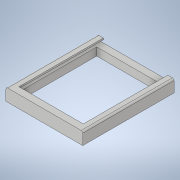
# Autodesk Inventor part: top_bracket_for_5mm
Saved by Autodesk Inventor 2020 (Build 240168000, 168)
## iProperties
Created: 2019-05-08
Part Number: top_bracket_for_5mm
Material: Generic
Document SubType Name: Modeling
Designer: aonih
Density: 1 g/cm^3
Appearance: Default
Author: aonih
Autodesk Inventor part; units mm, degrees
ref_plane "YZ Plane" through (0, 0, 0) normal (1, 0, 0) x (0, 1, 0)
ref_plane "XZ Plane" through (0, 0, 0) normal (0, 1, 0) x (-1, 0, 0)
ref_plane "XY Plane" through (0, 0, 0) normal (0, 0, 1) x (1, 0, 0)
sketch "Sketch1" plane through (0, 0, 0) normal (0, 1, 0) x (-1, 0, 0)
  line L0 (-71.5, -85) -> (71.5, -85)
  line L1 (71.5, -85) -> (71.5, 85)
  line L2 (71.5, 85) -> (-71.5, 85)
  line L3 (-71.5, 85) -> (-71.5, -85)
  line L4 (-71.5, -85) -> (71.5, 85) construction
  line L5 (71.5, -85) -> (-71.5, 85) construction
  point P0 (0, 0)
  dimension "d0" = 143
  dimension "d1" = 170
  constraints: 12 end point, 2 midpoint, 2 parallel, 1 horizontal, 1 perpendicular
  measures "d0" distance of L2.end L1.end
  measures "d1" distance of L1.end L0.end
extrude "Base" add sketch "Sketch1" along normal blind 23
sketch "Sketch2" plane through (0, 0, 0) normal (0, -1, 0) x (1, 0, 0)
  line L0 (-60, -72.5) -> (60, -72.5)
  line L1 (60, -72.5) -> (60, 72.5)
  line L2 (60, 72.5) -> (-60, 72.5)
  line L3 (-60, 72.5) -> (-60, -72.5)
  line L4 (-60, -72.5) -> (60, 72.5) construction
  line L5 (60, -72.5) -> (-60, 72.5) construction
  point P0 (0, 0)
  dimension "d4" = 120
  dimension "d5" = 145
  constraints: 12 end point, 2 midpoint, 2 parallel, 1 horizontal, 1 perpendicular
  measures "d4" distance of L2.end L1.end
  measures "d5" distance of L1.end L0.end
extrude "Extrusion2" cut sketch "Sketch2" against normal through all
sketch "Sketch3" plane through (0, 0, 0) normal (0, -1, 0) x (1, 0, 0)
  line L0 (63.65, -75.5) -> (-63.65, -75.5)
  line L1 (-63.65, -75.5) -> (-63.65, 75.5)
  line L2 (-63.65, 75.5) -> (63.65, 75.5)
  line L3 (63.65, 75.5) -> (63.65, -75.5)
  line L4 (-60, 72.5) -> (60, 72.5) projected
  line L5 (-60, -72.5) -> (-60, 72.5) projected
  line L6 (68.85, -80.7) -> (-68.85, -80.7)
  line L7 (-68.85, -80.7) -> (-68.85, 80.7)
  line L8 (-68.85, 80.7) -> (68.85, 80.7)
  line L9 (68.85, 80.7) -> (68.85, -80.7)
  line L10 (-71.5, 85) -> (71.5, 85) projected
  point P0 (0, 0)
  point P1 (63.65, 0)
  point P2 (68.85, 0)
  dimension "d9" = 3.65
  dimension "d10" = 5.2
  dimension "d11" = 12.5
  dimension "d38" = 5.2
  dimension "d39" = 151
  constraints: 16 end point, 4 parallel, 2 horizontal, 2 horizontal alignment, 2 midpoint, 2 perpendicular
  measures "d9" distance between parallel lines of L5 L1
  measures "d10" distance between parallel lines of L2 L8
  measures "d11" distance between parallel lines of L10 L4
  measures "d38" distance between parallel lines of L3 L9
  measures "d39" distance between parallel lines of L0 L2
extrude "Extrusion3" cut sketch "Sketch3" against normal blind 12
sketch "Sketch4" plane through (0, 12, 0) normal (0, -1, 0) x (1, 0, 0)
  line L0 (-68.85, 80.7) -> (68.85, 80.7) projected
  line L1 (63.65, 75.5) -> (-63.65, 75.5) projected
  line L2 (-53.85, 80.7) -> (-41.85, 80.7)
  line L3 (-41.85, 80.7) -> (-41.85, 75.5)
  line L4 (-41.85, 75.5) -> (-53.85, 75.5)
  line L5 (-53.85, 75.5) -> (-53.85, 80.7)
  line L6 (-68.85, -80.7) -> (-68.85, 80.7) projected
  line L7 (-63.65, 75.5) -> (-63.65, -75.5) projected
  line L8 (-63.65, 66.4) -> (-68.85, 66.4)
  line L9 (-68.85, 66.4) -> (-68.85, 54.4)
  line L10 (-68.85, 54.4) -> (-63.65, 54.4)
  line L11 (-63.65, 54.4) -> (-63.65, 66.4)
  line L12 (63.65, -75.5) -> (63.65, 75.5) projected
  line L13 (68.85, 80.7) -> (68.85, -80.7) projected
  line L14 (63.65, 66.4) -> (68.85, 66.4)
  line L15 (68.85, 66.4) -> (68.85, 54.4)
  line L16 (68.85, 54.4) -> (63.65, 54.4)
  line L17 (63.65, 54.4) -> (63.65, 66.4)
  line L18 (-63.65, -75.5) -> (63.65, -75.5) projected
  line L19 (68.85, -80.7) -> (-68.85, -80.7) projected
  line L20 (-53.85, -75.5) -> (-41.85, -75.5)
  line L21 (-41.85, -75.5) -> (-41.85, -80.7)
  line L22 (-41.85, -80.7) -> (-53.85, -80.7)
  line L23 (-53.85, -80.7) -> (-53.85, -75.5)
  line L24 (-68.85, -66.4) -> (-63.65, -66.4)
  line L25 (-63.65, -66.4) -> (-63.65, -54.4)
  line L26 (-63.65, -54.4) -> (-68.85, -54.4)
  line L27 (-68.85, -54.4) -> (-68.85, -66.4)
  line L28 (53.85, -80.7) -> (41.85, -80.7)
  line L29 (41.85, -80.7) -> (41.85, -75.5)
  line L30 (41.85, -75.5) -> (53.85, -75.5)
  line L31 (53.85, -75.5) -> (53.85, -80.7)
  line L32 (68.85, -54.4) -> (63.65, -54.4)
  line L33 (63.65, -54.4) -> (63.65, -66.4)
  line L34 (63.65, -66.4) -> (68.85, -66.4)
  line L35 (68.85, -66.4) -> (68.85, -54.4)
  line L36 (53.85, 75.5) -> (41.85, 75.5)
  line L37 (41.85, 75.5) -> (41.85, 80.7)
  line L38 (41.85, 80.7) -> (53.85, 80.7)
  line L39 (53.85, 80.7) -> (53.85, 75.5)
  point P0 (0, 0)
  point P1 (66.25, 66.4)
  point P2 (-66.25, 66.4)
  point P3 (-53.85, -78.1)
  point P4 (-53.85, 78.1)
  point P5 (66.25, -54.4)
  point P6 (-66.25, -54.4)
  point P7 (41.85, 78.1)
  point P8 (41.85, -78.1)
  dimension "d14" = 12
  dimension "d15" = 15
  dimension "d16" = 12
  dimension "d17" = 14.3
  dimension "d18" = 12
  dimension "d19" = 12
  dimension "d20" = 14.3
  dimension "d21" = 12
  dimension "d22" = 12
  dimension "d23" = 15
  dimension "d24" = 12
  dimension "d25" = 12
  constraints: 64 end point, 16 parallel, 16 point on line, 8 horizontal, 8 midpoint, 8 perpendicular, 2 horizontal alignment, 2 vertical alignment
  measures "d14" distance between parallel lines of L3 L5
  measures "d15" distance between parallel lines of L6 L5
  measures "d16" distance between parallel lines of L8 L10
  measures "d17" distance between parallel lines of L0 L8
  measures "d18" distance between parallel lines of L14 L16
  measures "d19" distance between parallel lines of L21 L23
  measures "d20" distance between parallel lines of L19 L24
  measures "d21" distance between parallel lines of L26 L24
  measures "d22" distance between parallel lines of L34 L32
  measures "d23" distance between parallel lines of L13 L31
  measures "d24" distance between parallel lines of L31 L29
  measures "d25" distance between parallel lines of L39 L37
extrude "Extrusion4" add sketch "Sketch4" along normal blind 7 contours L0 L3 L1 L5 | L8 L7 L10 L6 | L0 L39 L1 L37 | L26 L7 L24 L6 | L13 L16 L12 L14 | L23 L18 L21 L19 | L13 L34 L12 L32 | L29 L18 L31 L19
fillet "Fillet1" radius 1.25 16 edges at (-66.25, 5, 54.4) (-66.25, 5, 66.4) (-66.25, 5, -66.4) (-66.25, 5, -54.4) (66.25, 5, -66.4) (66.25, 5, -54.4) (66.25, 5, 54.4) (66.25, 5, 66.4) (53.85, 5, -78.1) (41.85, 5, -78.1) (-53.85, 5, -78.1) (-41.85, 5, -78.1) (-53.85, 5, 78.1) (-41.85, 5, 78.1) (41.85, 5, 78.1) (53.85, 5, 78.1)
sketch "Sketch5" plane through (71.5, 0, -85) normal (0, 0, -1) x (-1, 0, 0)
  line L0 (71.5, 0) -> (71.5, 23) construction
  line L1 (131.5, 23) -> (11.5, 23) construction
  line L2 (5, 20.05) -> (138, 20.05)
  line L3 (138, 20.05) -> (138, 14.8)
  line L4 (138, 14.8) -> (5, 14.8)
  line L5 (5, 14.8) -> (5, 20.05)
  line L6 (0, 0) -> (143, 0) projected
  point P0 (71.5, 20.05)
  dimension "d29" = 133
  dimension "d30" = 5.25
  dimension "d31" = 14.8
  constraints: 10 end point, 2 midpoint, 2 parallel, 1 horizontal, 1 perpendicular, 1 point on line
  measures "d29" distance of L3.end L4.end
  measures "d30" distance of L2.end L3.end
  measures "d31" distance between parallel lines of L6 L4
extrude "Extrusion5" cut sketch "Sketch5" against normal blind 165
fillet "Fillet2" radius 3 2 edges at (71.5, 23, 0) (-71.5, 23, 0)
sketch "Sketch6" plane through (71.5, 0, -85) normal (0, 0, -1) x (-1, 0, 0)
  line L0 (3, 23) -> (140, 23) projected
  line L1 (5, 20.05) -> (138, 20.05) projected
  line L2 (11.5, 23) -> (131.5, 23)
  line L3 (131.5, 23) -> (131.5, 20.05)
  line L4 (131.5, 20.05) -> (11.5, 20.05)
  line L5 (11.5, 20.05) -> (11.5, 23)
  line L6 (0, 0) -> (143, 0) construction
  point P0 (71.5, 0)
  point P1 (71.5, 23)
  point P2 (71.5, 0)
  dimension "d35" = 120
  constraints: 8 end point, 2 midpoint, 2 parallel, 2 point on line, 1 horizontal, 1 perpendicular, 1 vertical alignment
  measures "d35" distance between parallel lines of L3 L5
extrude "Extrusion6" cut sketch "Sketch6" against normal blind 12.5
equation "\"d9\" = d8"
equation "\"d16\" = d14"
equation "\"d18\" = d14"
equation "\"d19\" = d14"
equation "\"d20\" = d17"
equation "\"d21\" = d19"
equation "\"d22\" = d14"
equation "\"d23\" = d15"
equation "\"d24\" = d14"
equation "\"d8\" = -0.5 * d10 + 0.5 * d11"
body "Solid1"
